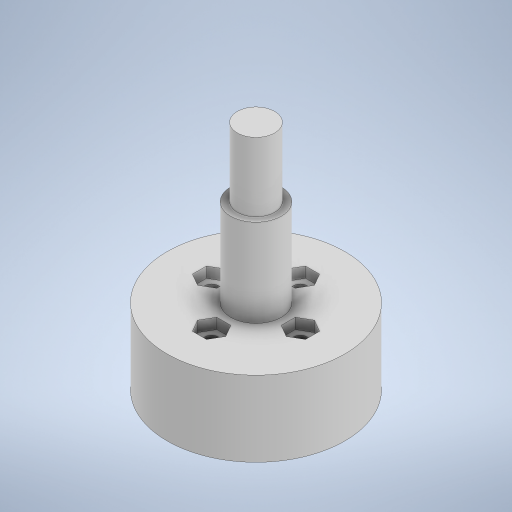
# Autodesk Inventor part: Encoder_coupler
Saved by Autodesk Inventor 2024.2 (Build 282272000, 272)
## iProperties
Created: 2024-05-10
Part Number: Encoder_coupler
Material: Generic
Document SubType Name: Modeling
Designer: tamiz
Density: 1 g/cm^3
Appearance: Default
Author: tamiz
## iProperties of the stored document Encoder_coupler_3DPrint.ipt
Created: 2024-05-10
Part Number: Encoder_coupler_3DPrint
Material: Generic
Document SubType Name: Modeling
Designer: tamiz
Density: 1 g/cm^3
Appearance: Default
Author: tamiz
Autodesk Inventor part; units mm, degrees
ref_plane "YZ Plane" through (0, 0, 0) normal (1, 0, 0) x (0, 1, 0)
ref_plane "XZ Plane" through (0, 0, 0) normal (0, 1, 0) x (-1, 0, 0)
ref_plane "XY Plane" through (0, 0, 0) normal (0, 0, 1) x (1, 0, 0)
sketch "Sketch1" plane through (0, 0, 0) normal (0, 1, 0) x (-1, 0, 0)
  circle A0 centre (0, 0) radius 20
  dimension "d0" = 40
  constraints: 1 centre point, 1 coincident
  measures "d0" diameter of A0
extrude "Extrusion1" add sketch "Sketch1" along normal blind 17
sketch "Sketch2" plane through (0, 17, 0) normal (0, 1, 0) x (1, 0, 0)
  circle A0 centre (-10, 0) radius 1.5
  circle A1 centre (10, 0) radius 1.5
  circle A2 centre (0, 10) radius 1.5
  circle A3 centre (0, -10) radius 1.5
  circle A4 centre (0, 0) radius 4.2
  circle A5 centre (0, 0) radius 5.7
  line L0 (-10, 3.1754) -> (-7.25, 1.5877)
  line L1 (-7.25, 1.5877) -> (-7.25, -1.5877)
  line L2 (-7.25, -1.5877) -> (-10, -3.1754)
  line L3 (-10, -3.1754) -> (-12.75, -1.5877)
  line L4 (-12.75, -1.5877) -> (-12.75, 1.5877)
  line L5 (-12.75, 1.5877) -> (-10, 3.1754)
  line L6 (10, 3.1754) -> (7.25, 1.5877)
  line L7 (7.25, 1.5877) -> (7.25, -1.5877)
  line L8 (7.25, -1.5877) -> (10, -3.1754)
  line L9 (10, -3.1754) -> (12.75, -1.5877)
  line L10 (12.75, -1.5877) -> (12.75, 1.5877)
  line L11 (12.75, 1.5877) -> (10, 3.1754)
  line L12 (1.5877, 12.75) -> (3.1754, 10)
  line L13 (-1.5877, 12.75) -> (1.5877, 12.75)
  line L14 (-3.1754, 10) -> (-1.5877, 12.75)
  line L15 (-1.5877, 7.25) -> (-3.1754, 10)
  line L16 (1.5877, 7.25) -> (-1.5877, 7.25)
  line L17 (3.1754, 10) -> (1.5877, 7.25)
  line L18 (3.1754, -10) -> (1.5877, -7.25)
  line L19 (1.5877, -12.75) -> (3.1754, -10)
  line L20 (-1.5877, -12.75) -> (1.5877, -12.75)
  line L21 (-3.1754, -10) -> (-1.5877, -12.75)
  line L22 (-1.5877, -7.25) -> (-3.1754, -10)
  line L23 (1.5877, -7.25) -> (-1.5877, -7.25)
  dimension "d6" = 3
  dimension "d13" = 8.4
  dimension "d16" = 1.5
  constraints: 48 end point, 6 centre point
  measures "d6" diameter of A1
  measures "d13" diameter of A4
  measures "d16" radial gap between concentric circles of A4 A5
sketch "Sketch3" plane through (0, 0, 0) normal (0, -1, 0) x (1, 0, 0)
  circle A0 centre (0, 0) radius 3.5
  dimension "d8" = 7
  constraints: 1 centre point, 1 coincident
  measures "d8" diameter of A0
extrude "Extrusion2" cut sketch "Sketch3" against normal blind 5
extrude "Extrusion4" cut sketch "Sketch2" against normal through all contours A0 | A1 | A2 | A3
extrude "Extrusion5" add sketch "Sketch2" along normal blind 19.75 contours A5
extrude "Extrusion6" add sketch "Sketch2" along normal blind 35.25 contours A4
extrude "Extrusion7" cut sketch "Sketch2" against normal blind 2.4 contours A0 | L0 L1 L2 L3 L4 L5 | L11 L10 L9 L8 L7 L6 | L12 L17 L16 L15 L14 L13 | L19 L20 L21 L22 L23 L18
body "Solid1"
